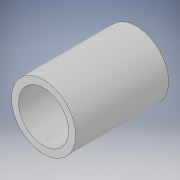
# Autodesk Inventor part: Parts_CoilSpring_CP_0.5-4.5-6.5
Saved by Autodesk Inventor 2019.1 (Build 231200000, 200)
## iProperties
Created: 2018-08-20
Part Number: Parts_CoilSpring_CP_0.5-4.5-6.5
Material: Generic
Document SubType Name: Modeling
Designer: sktom
Density: 1 g/cm^3
Appearance: Default
Author: sktom
Autodesk Inventor part; units mm, degrees
ref_plane "YZ Plane" through (0, 0, 0) normal (1, 0, 0) x (0, 1, 0)
ref_plane "XZ Plane" through (0, 0, 0) normal (0, 1, 0) x (-1, 0, 0)
ref_plane "XY Plane" through (0, 0, 0) normal (0, 0, 1) x (1, 0, 0)
sketch "スケッチ1" plane through (0, 0, 0) normal (0, 0, 1) x (1, 0, 0)
  circle A0 centre (0, 0) radius 2.25
  circle A1 centre (0, 0) radius 1.75
  dimension "d0" = 4.5
  dimension "d4" = 0.5
  constraints: 2 centre point, 1 coincident
  measures "d0" diameter of A0
  measures "d4" radial gap between concentric circles of A0 A1
extrude "押し出し2" add sketch "スケッチ1" along normal blind 6.5
